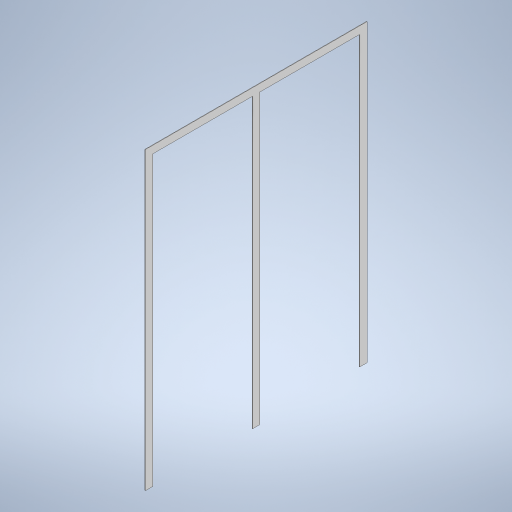
# Autodesk Inventor part: shelf
Saved by Autodesk Inventor 2023 (Build 270158000, 158)
## iProperties
Created: 2022-06-10
Part Number: shelf
Material: Generisch
Document SubType Name: Modeling
Designer: Tim Stechel
Density: 1 g/cm^3
Appearance: Vorgabe
Author: Tim Stechel
Autodesk Inventor part; units mm, degrees
ref_plane "YZ Plane" through (0, 0, 0) normal (1, 0, 0) x (0, 1, 0)
ref_plane "XZ Plane" through (0, 0, 0) normal (0, 1, 0) x (-1, 0, 0)
ref_plane "XY Plane" through (0, 0, 0) normal (0, 0, 1) x (1, 0, 0)
sketch "Skizze1" plane through (0, 0, 0) normal (1, 0, 0) x (0, 1, 0)
  line L0 (0, -3.0223) -> (0, -427.4276)
  line L1 (0, 0) -> (600, 0)
  line L2 (600, 0) -> (600, -450)
  line L3 (600, -450) -> (0, -450)
  line L4 (0, -450) -> (0, 0)
  line L5 (600, 0) -> (585, 0)
  line L6 (585, 0) -> (585, -450)
  line L7 (0, 0) -> (15, 0)
  line L8 (585, 0) -> (585, -15)
  line L9 (585, -15) -> (15, -15)
  line L10 (585, -225) -> (585, -217.5)
  line L11 (585, -217.5) -> (585, -232.5)
  line L12 (585, -232.5) -> (15, -232.5)
  line L13 (585, -217.5) -> (15, -217.5)
  line L14 (585, -450) -> (585, -435)
  line L15 (585, -435) -> (15, -435)
  line L16 (585, -232.5) -> (585, -240)
  line L17 (555, -240) -> (555, -270)
  line L18 (554.8716, -281.2484) -> (554.8716, -311.2484)
  line L19 (554.8716, -321.2484) -> (554.8716, -351.2484)
  line L20 (554.8716, -358.8081) -> (554.8716, -388.8081)
  line L21 (554.8716, -398.5513) -> (554.8716, -428.5513)
  line L22 (564.8716, -321.2484) -> (564.8716, -351.2484)
  line L23 (565, -240) -> (565, -270)
  line L24 (564.8716, -281.2484) -> (564.8716, -311.2484)
  line L25 (564.8716, -358.8081) -> (564.8716, -388.8081)
  line L26 (564.8716, -398.5513) -> (564.8716, -428.5513)
  line L27 (574.8716, -321.2484) -> (574.8716, -351.2484)
  line L28 (575, -240) -> (575, -270)
  line L29 (574.8716, -281.2484) -> (574.8716, -311.2484)
  line L30 (574.8716, -358.8081) -> (574.8716, -388.8081)
  line L31 (574.8716, -398.5513) -> (574.8716, -428.5513)
  line L32 (570.1874, -253.3785) -> (570.1874, -288.3785)
  line L33 (570.1874, -298.063) -> (570.1874, -333.063)
  line L34 (570.1874, -341.7513) -> (570.1874, -371.7513)
  line L35 (570.1874, -382.1768) -> (570.1874, -417.1768)
  line L36 (560.1874, -382.1768) -> (560.1874, -417.1768)
  line L37 (560.1874, -341.7513) -> (560.1874, -371.7513)
  line L38 (560.1874, -298.063) -> (560.1874, -333.063)
  line L39 (560.1874, -253.3785) -> (560.1874, -288.3785)
  line L40 (585, -15) -> (15, -15)
  line L41 (554.8716, -181.0513) -> (554.8716, -211.0513)
  line L42 (560.1874, -164.6768) -> (560.1874, -199.6768)
  line L43 (564.8716, -181.0513) -> (564.8716, -211.0513)
  line L44 (570.1874, -164.6768) -> (570.1874, -199.6768)
  line L45 (574.8716, -181.0513) -> (574.8716, -211.0513)
  line L46 (554.8716, -103.7484) -> (554.8716, -133.7484)
  line L47 (554.8716, -141.3081) -> (554.8716, -171.3081)
  line L48 (564.8716, -103.7484) -> (564.8716, -133.7484)
  line L49 (560.1874, -124.2513) -> (560.1874, -154.2513)
  line L50 (570.1874, -124.2513) -> (570.1874, -154.2513)
  line L51 (564.8716, -141.3081) -> (564.8716, -171.3081)
  line L52 (574.8716, -141.3081) -> (574.8716, -171.3081)
  line L53 (574.8716, -103.7484) -> (574.8716, -133.7484)
  line L54 (555, -22.5) -> (555, -52.5)
  line L55 (554.8716, -63.7484) -> (554.8716, -93.7484)
  line L56 (565, -22.5) -> (565, -52.5)
  line L57 (560.1874, -80.563) -> (560.1874, -115.563)
  line L58 (570.1874, -80.563) -> (570.1874, -115.563)
  line L59 (564.8716, -63.7484) -> (564.8716, -93.7484)
  line L60 (574.8716, -63.7484) -> (574.8716, -93.7484)
  line L61 (560.1874, -35.8785) -> (560.1874, -70.8785)
  line L62 (570.1874, -35.8785) -> (570.1874, -70.8785)
  line L63 (575, -22.5) -> (575, -52.5)
  line L64 (15, -15) -> (0, -15)
  line L65 (15, -217.5) -> (0, -217.5)
  line L66 (15, -232.5) -> (0, -232.5)
  line L67 (15, -435) -> (0, -435)
  line L68 (600, -15) -> (300, -15)
  line L69 (300, -15) -> (300, -217.5)
  line L70 (300, -232.5) -> (300, -435)
  line L71 (285, -217.5) -> (-285, -217.5)
  line L72 (285, -232.5) -> (-285, -232.5)
  line L73 (264.8716, -63.7484) -> (264.8716, -93.7484)
  line L74 (260.1874, -35.8785) -> (260.1874, -70.8785)
  line L75 (255, -22.5) -> (255, -52.5)
  line L76 (254.8716, -63.7484) -> (254.8716, -93.7484)
  line L77 (274.8716, -358.8081) -> (274.8716, -388.8081)
  line L78 (264.8716, -358.8081) -> (264.8716, -388.8081)
  line L79 (254.8716, -358.8081) -> (254.8716, -388.8081)
  line L80 (270.1874, -341.7513) -> (270.1874, -371.7513)
  line L81 (260.1874, -341.7513) -> (260.1874, -371.7513)
  line L82 (260.1874, -298.063) -> (260.1874, -333.063)
  line L83 (270.1874, -298.063) -> (270.1874, -333.063)
  line L84 (254.8716, -321.2484) -> (254.8716, -351.2484)
  line L85 (264.8716, -321.2484) -> (264.8716, -351.2484)
  line L86 (274.8716, -321.2484) -> (274.8716, -351.2484)
  line L87 (255, -240) -> (255, -270)
  line L88 (254.8716, -281.2484) -> (254.8716, -311.2484)
  line L89 (264.8716, -281.2484) -> (264.8716, -311.2484)
  line L90 (274.8716, -281.2484) -> (274.8716, -311.2484)
  line L91 (270.1874, -253.3785) -> (270.1874, -288.3785)
  line L92 (260.1874, -253.3785) -> (260.1874, -288.3785)
  line L93 (275, -240) -> (275, -270)
  line L94 (265, -240) -> (265, -270)
  line L95 (270.1874, -382.1768) -> (270.1874, -417.1768)
  line L96 (260.1874, -382.1768) -> (260.1874, -417.1768)
  line L97 (254.8716, -398.5513) -> (254.8716, -428.5513)
  line L98 (264.8716, -398.5513) -> (264.8716, -428.5513)
  line L99 (274.8716, -398.5513) -> (274.8716, -428.5513)
  line L100 (254.8716, -103.7484) -> (254.8716, -133.7484)
  line L101 (254.8716, -141.3081) -> (254.8716, -171.3081)
  line L102 (260.1874, -80.563) -> (260.1874, -115.563)
  line L103 (270.1874, -80.563) -> (270.1874, -115.563)
  line L104 (264.8716, -103.7484) -> (264.8716, -133.7484)
  line L105 (260.1874, -124.2513) -> (260.1874, -154.2513)
  line L106 (270.1874, -124.2513) -> (270.1874, -154.2513)
  line L107 (264.8716, -141.3081) -> (264.8716, -171.3081)
  line L108 (274.8716, -63.7484) -> (274.8716, -93.7484)
  line L109 (270.1874, -35.8785) -> (270.1874, -70.8785)
  line L110 (275, -22.5) -> (275, -52.5)
  line L111 (264.8716, -181.0513) -> (264.8716, -211.0513)
  line L112 (274.8716, -181.0513) -> (274.8716, -211.0513)
  line L113 (254.8716, -181.0513) -> (254.8716, -211.0513)
  line L114 (260.1874, -164.6768) -> (260.1874, -199.6768)
  line L115 (270.1874, -164.6768) -> (270.1874, -199.6768)
  line L116 (274.8716, -141.3081) -> (274.8716, -171.3081)
  line L117 (274.8716, -103.7484) -> (274.8716, -133.7484)
  line L118 (265, -22.5) -> (265, -52.5)
  point P0 (0, -217.5)
  point P1 (0, -232.5)
  point P2 (0, -15)
  point P3 (0, -217.5)
  point P4 (0, -232.5)
  dimension "d0" = 450
  dimension "d1" = 600
  dimension "d2" = 15
  dimension "d3" = 450
  dimension "d4" = 15
  dimension "d6" = 15
  dimension "d9" = 7.5
  dimension "d10" = 15
  dimension "d11" = 15
  dimension "d12" = 7.5
  dimension "d13" = 30
  dimension "d14" = 30
  dimension "d24" = 30
  dimension "d25" = 10
  dimension "d26" = 30
  dimension "d28" = 30
  dimension "d30" = 30
  dimension "d33" = 10
  dimension "d40" = 35
  dimension "d42" = 30
  dimension "d44" = 35
  dimension "d45" = 35
  dimension "d48" = 10
  dimension "d55" = 217.5
  dimension "d60" = 300
  dimension "d63" = 300
  constraints: 238 end point, 54 point on line, 5 horizontal, 5 midpoint, 5 parallel, 5 vertical, 2 perpendicular, 1 collinear, 259 other
  measures "d0" distance of L1.end L2.end
  measures "d1" distance of L2.end L3.end
  measures "d2" distance of L1.end L5.end
  measures "d3" distance of L5.end L6.end
  measures "d4" distance of L1.start L7.end
  measures "d6" distance of L5.end L8.end
  measures "d9" distance of L10.start L10.end
  measures "d10" distance of L10.end L11.end
  measures "d11" distance of L6.end L14.end
  measures "d12" distance of L11.end L16.end
  measures "d13" distance of L16.end L17.start
  measures "d14" distance of L17.start L17.end
  measures "d24" distance of L18.start L18.end
  measures "d25" distance of L18.end L19.start
  measures "d26" distance of L19.start L19.end
  measures "d28" distance of L20.start L20.end
  measures "d30" distance of L21.start L21.end
  measures "d33" distance of L19.start L22.start
  measures "d40" distance of L33.start L33.end
  measures "d42" distance of L34.start L34.end
  measures "d44" distance of L35.start L35.end
  measures "d45" distance of L32.start L32.end
  measures "d48" distance of L35.start L36.start
  measures "d55" distance of L11.end L40.start
  measures "d60" distance of L68.start L68.end
  measures "d63" distance of L58.start L103.start
extrude "Extrusion1" add sketch "Skizze1" along normal blind 1 contours L4 L1 L6 L9 L64 L0 | L65 L13 L6 L12 L66 L0 | L1 L2 L68 L6 | L68 L2 L3 L6 | L67 L15 L6 L3 L4
equation "\"d3\" = d0"
